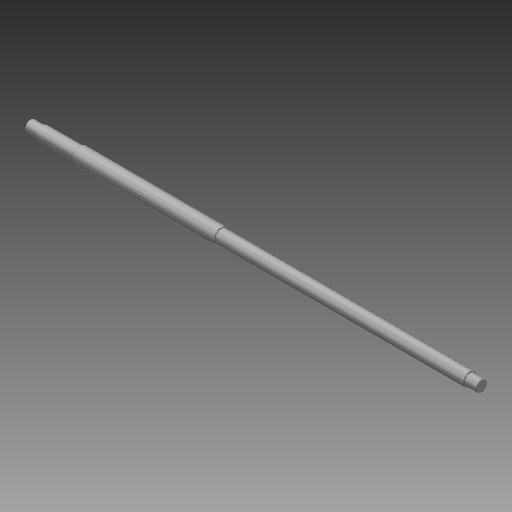
# Autodesk Inventor part: Eje
Saved by Autodesk Inventor 2019 (Build 230136000, 136)
## iProperties
Created: 2019-11-15
Part Number: Eje
Material: Steel
Document SubType Name: Modeling
Designer: eddysanoli
Density: 1 g/cm^3
Appearance: Steel
CustomPartVersion: 1
Author: eddysanoli
Autodesk Inventor part; units mm, degrees
ref_plane "Plano inicial" through (0, 0, 0) normal (1, 0, 0) x (0, 1, 0)
ref_plane "XZ Plane" through (0, 0, 0) normal (0, 1, 0) x (-1, 0, 0)
ref_plane "XY Plane" through (0, 0, 0) normal (0, 0, 1) x (1, 0, 0)
sketch "Boceto principal" plane through (0, 0, 0) normal (0, 0, 1) x (1, 0, 0)
  line L0 (0, 0) -> (440.47, 0)
  line L1 (11.5, 5.5) -> (11.5, 6.5)
  line L2 (11.5, 6.5) -> (48.5, 6.5)
  line L3 (0, 5.5) -> (11.5, 5.5)
  line L4 (186.707, 7.5) -> (186.707, 6.5)
  line L5 (48.5, 7.5) -> (186.707, 7.5)
  line L6 (0, 0) -> (0, 5.5)
  line L7 (48.5, 6.5) -> (48.5, 7.5)
  line L8 (186.707, 6.5) -> (207, 6.5)
  line L9 (207, 6.5) -> (287.1, 6.5)
  line L10 (287.1, 6.5) -> (391.97, 6.5)
  line L11 (428.97, 6.5) -> (428.97, 5.5)
  line L12 (391.97, 6.5) -> (428.97, 6.5)
  line L13 (440.47, 5.5) -> (440.47, 0)
  line L14 (428.97, 5.5) -> (440.47, 5.5)
  dimension "d3" = 13
  dimension "d4" = 11
  dimension "d5" = 15
  dimension "d10" = 13
  dimension "d11" = 13
  dimension "d12" = 13
  dimension "d13" = 13
  dimension "d41" = 11
  constraints: 30 end point, 6 vertical, 3 horizontal
  measures "d3" diameter of L2 L0
  measures "d4" diameter of L3 L0
  measures "d5" diameter of L5 L0
  measures "d10" diameter of L8 L0
  measures "d11" diameter of L9 L0
  measures "d12" diameter of L10 L0
  measures "d13" diameter of L12 L0
  measures "d41" diameter of L14 L0
revolve "Revolución1" add sketch "Boceto principal" angle 360 about axis through (0, 0, 0) along (1, 0, 0)
fillet "Fillet7" radius 0.5 1 edges at (428.97, -5.5, 0)
chamfer "Chamfer9" distance 0.5 angle 45 1 edges at (440.47, -5.5, 0) measured on face at (433.1367, 5.4288, -0.8823)
chamfer "Chamfer2" distance 0.5 angle 45 1 edges at (0, -5.5, 0) measured on face at (3.8333, 5.4288, -0.8823)
fillet "Fillet1" radius 0.5 1 edges at (11.5, -5.5, 0)
fillet "Fillet2" radius 0.5 1 edges at (48.5, -6.5, 0)
chamfer "Chamfer3" distance 0.5 angle 45 1 edges at (48.5, -7.5, 0) measured on face at (94.569, 7.4029, -1.2031)
chamfer "Chamfer4" distance 0.5 angle 45 1 edges at (186.707, -7.5, 0) measured on face at (94.9023, 7.4757, -0.6035)
fillet "Fillet3" radius 0.5 1 edges at (186.707, -6.5, 0)
chamfer "Chamfer8" distance 0.5 angle 45 1 edges at (428.97, -6.5, 0) measured on face at (404.3033, 6.4158, -1.0427)
chamfer "Chaflán1" distance 0.5 angle 45 1 edges at (11.5, -6.5, 0) measured on face at (23.6667, 6.4789, -0.523)
